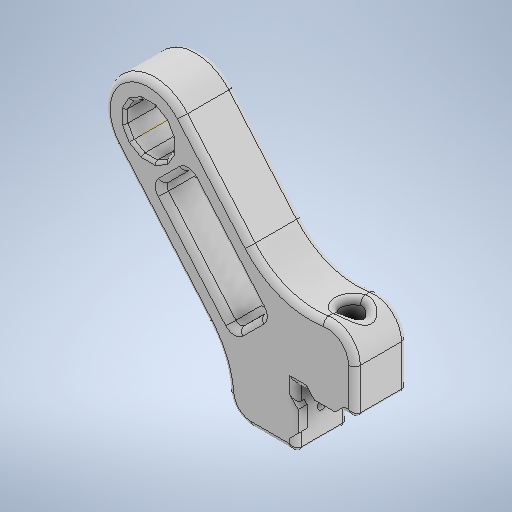
# Autodesk Inventor part: Z-Endstop
Saved by Autodesk Inventor 2025.3 (Build 293356030, 356C)
## iProperties
Created: 2025-10-01
Part Number: Z-Endstop
Material: Generic
Document SubType Name: Modeling
Designer: tvoko
Density: 1 g/cm^3
Appearance: Default
Author: tvoko
Autodesk Inventor part; units mm, degrees
ref_plane "YZ Plane" through (0, 0, 0) normal (1, 0, 0) x (0, 1, 0)
ref_plane "XZ Plane" through (0, 0, 0) normal (0, 1, 0) x (-1, 0, 0)
ref_plane "XY Plane" through (0, 0, 0) normal (0, 0, 1) x (1, 0, 0)
sketch "Sketch1" plane through (0, 0, 0) normal (0, 0, 1) x (1, 0, 0)
  line L0 (-10.05, 10.05) -> (10.05, 10.05)
  line L1 (10.05, 10.05) -> (10.05, -10.05)
  line L2 (10.05, -10.05) -> (-10.05, -10.05)
  line L3 (-10.05, -10.05) -> (-10.05, 10.05)
  line L4 (0, 10.05) -> (0, -10.05) construction
  line L5 (-10.05, 0) -> (10.05, 0) construction
  line L6 (-10.05, 4.5) -> (-9.05, 3.5)
  line L7 (-9.05, 3.5) -> (-9.05, -3.5)
  line L8 (-9.05, -3.5) -> (-10.05, -4.5)
  line L9 (-4.5, 10.05) -> (-3.5, 9.05)
  line L10 (-3.5, 9.05) -> (3.5, 9.05)
  line L11 (3.5, 9.05) -> (4.5, 10.05)
  line L12 (10.05, 10.05) -> (10.05, 25.05)
  line L13 (-10.05, -10.05) -> (-25.05, -10.05)
  line L14 (-25.05, -10.05) -> (-25.05, 10.05)
  line L15 (-9.95, 25.05) -> (-25.05, 10.05)
  line L16 (10.05, 25.05) -> (-9.95, 25.05)
  line L17 (-9.95, 25.05) -> (-9.95, 10.05)
  line L18 (-10.05, 9.95) -> (-25.05, 9.95)
  circle A0 centre (-60, 60) radius 7.95 construction
  arc A1 (-48.653453, 69.811007) -> (-71.346547, 50.188993) centre (-60, 60) ccw
  line L19 (-48.653453, 69.811007) -> (-25.647611, 43.204476)
  line L20 (-71.346547, 50.188993) -> (-39.889181, 13.808171)
  line L21 (-31.969587, 6.010347) -> (-25.05, -10.05) construction
  line L22 (-9.95, 25.05) -> (-31.969587, 6.010347) construction
  line L23 (-9.95, 25.05) -> (-0.739164, 34.199837) construction
  arc A2 (10.05, 25.05) -> (-0.739164, 34.199837) centre (0.775622, 25.05) ccw
  arc A3 (-25.647611, 43.204476) -> (-0.739164, 34.199837) centre (-5.162352, 60.917444) ccw
  line L24 (-25.647611, 43.204476) -> (-9.95, 25.05) construction
  line L25 (-55.410065, 67.95) -> (-50.820131, 60)
  line L26 (-50.820131, 60) -> (-55.410065, 52.05)
  line L27 (-55.410065, 52.05) -> (-64.589935, 52.05)
  line L28 (-64.589935, 52.05) -> (-69.179869, 60)
  line L29 (-69.179869, 60) -> (-64.589935, 67.95)
  line L30 (-64.589935, 67.95) -> (-55.410065, 67.95)
  line L31 (-60, 69.179869) -> (-52.05, 64.589935)
  line L32 (-52.05, 64.589935) -> (-52.05, 55.410065)
  line L33 (-52.05, 55.410065) -> (-60, 50.820131)
  line L34 (-60, 50.820131) -> (-67.95, 55.410065)
  line L35 (-67.95, 55.410065) -> (-67.95, 64.589935)
  line L36 (-67.95, 64.589935) -> (-60, 69.179869)
  line L37 (-47.974498, 53.52563) -> (-55.086003, 46.461221)
  line L38 (-55.189369, 43.734182) -> (-32.242214, 17.195522)
  line L39 (-29.319833, 17.084752) -> (-22.208328, 24.149161)
  line L40 (-22.104962, 26.8762) -> (-45.052118, 53.41486)
  arc A4 (-45.052118, 53.41486) -> (-47.974498, 53.52563) centre (-46.564991, 52.106726) ccw
  arc A5 (-22.208328, 24.149161) -> (-22.104962, 26.8762) centre (-23.617835, 25.568065) ccw
  arc A6 (-32.242214, 17.195522) -> (-29.319833, 17.084752) centre (-30.729341, 18.503656) ccw
  arc A7 (-55.086003, 46.461221) -> (-55.189369, 43.734182) centre (-53.676496, 45.042317) ccw
  arc A8 (-32.932093, -2.78299) -> (-39.889181, 13.808171) centre (-61.791846, -5.130384) ccw
  arc A9 (-32.932093, -2.78299) -> (-25.05, -10.05) centre (-25.05, -2.141876) ccw
  point P0 (0, 0)
  point P1 (0, 0)
  point P2 (0, 9.05)
  point P3 (-9.05, 0)
  point P4 (-60, 67.95)
  point P5 (-63.975, 66.884902)
  point P6 (-52.05, 62.130196)
  point P7 (-52.05, 57.869804)
  point P8 (-54.180196, 54.180196)
  point P9 (-57.869804, 52.05)
  point P10 (-62.130196, 52.05)
  point P11 (-65.819804, 54.180196)
  point P12 (-67.95, 57.869804)
  point P13 (-67.95, 62.130196)
  point P14 (-57.869804, 67.95)
  point P15 (-54.180196, 65.819804)
  point P16 (-65.819804, 65.819804)
  point P17 (-62.130196, 67.95)
  dimension "d0" = 20.1
  dimension "d1" = 7
  dimension "d2" = 1
  dimension "d3" = 135
  dimension "d4" = 1
  dimension "d5" = 7
  dimension "d6" = 135
  dimension "d8" = 15
  dimension "d9" = 15
  dimension "d18" = 20
  dimension "d19" = 20
  dimension "d62" = 60
  dimension "d63" = 15.9
  dimension "d64" = 30
  dimension "d65" = 24
  dimension "d72" = 2
  dimension "d73" = 8
  dimension "d75" = 8
  dimension "d76" = 8
  dimension "d77" = 39
  dimension "d80" = 60
  constraints: 83 end point, 20 point on circle, 16 tangent, 10 centre point, 9 midpoint, 9 point on line, 7 parallel, 7 perpendicular, 5 horizontal, 4 coincident, 4 equal length, 3 equal radius, 2 vertical, 1 collinear, 26 other
  measures "d0" distance of L0.start L0.end
  measures "d1" distance of L9.end L10.end
  measures "d2" distance between parallel lines of L0 L10
  measures "d3" angle of L10 L11
  measures "d4" distance between parallel lines of L3 L7
  measures "d5" distance of L6.end L7.end
  measures "d6" angle of L7 L6
  measures "d8" distance of L2.end L13.end
  measures "d9" distance of L0.end L12.end
  measures "d18" distance of L12.end L15.start
  measures "d19" distance between parallel lines of L13 L18
  measures "d62" distance from line of A0.centre L5
  measures "d63" diameter of A0
  measures "d64" diameter of A1
  measures "d65" distance of L19.end L15.start
  measures "d72" radius of A4
  measures "d73" distance between parallel lines of L19 L40
  measures "d75" distance between parallel lines of L20 L38
  measures "d76" distance between parallel lines of L15 L39
  measures "d77" distance between parallel lines of L39 L37
  measures "d80" distance from line of L4 A0.centre
extrude "Extrusion1" add sketch "Sketch1" along normal mid plane 18 contours L3 L18 L14 L15 L17 L0 | L17 L16 L12 L0 | L3 L13 L14 L18 | L0 L11 L10 L9 | L15 L14 A9 A8 L20 A1 L19 A3 A2 L16 | L6 L7 L8 L3 | L25 L31 L30 | L31 L32 L25 | L30 L36 L31 | L25 L26 L32 | L36 L29 L30 | L32 L33 L26 | L29 L35 L36 | L26 L27 L33 | L35 L28 L29 | L33 L34 L27 | L28 L34 L35 | L27 L28 L34
fillet "Fillet1" radius 1 2 edges at (10.05, 10.05, 0) (-10.05, -10.05, 0)
sketch "Sketch2" plane through (-4.5, 9.05, -9) normal (0, -1, 0) x (-1, 0, 0)
  line L0 (-9, -18) -> (-13.55, -18) projected
  line L1 (-9, 0) -> (-9, -18) projected
  line L2 (0, 0) -> (0, -18) projected
  circle A0 centre (-4.5, -9) radius 1.55
  circle A1 centre (-4.5, -9) radius 3.5
  line L3 (5.55, 0) -> (5.55, -18) projected
  line L4 (0, 0) -> (5.55, 0) projected
  line L5 (-8, 0) -> (-1, 0) projected
  line L6 (-13.55, 0) -> (-9, 0) projected
  line L7 (-13.55, -18) -> (-13.55, 0) projected
  line L8 (5.55, -18) -> (0, -18) projected
  line L9 (-9, -9) -> (0, -9) construction
  line L10 (-9, -15) -> (0, -15)
  line L11 (0, -15) -> (0, -3)
  line L12 (0, -3) -> (-9, -3)
  line L13 (-9, -3) -> (-9, -15)
  point P0 (-4.5, -9)
  point P1 (-1, 0)
  point P2 (0, -15)
  dimension "d26" = 3.1
  dimension "d27" = 7
  dimension "d66" = 12
  constraints: 10 end point, 4 midpoint, 2 centre point, 2 coincident, 2 parallel, 2 point on line, 1 horizontal, 1 perpendicular, 1 other
  measures "d26" diameter of A0
  measures "d27" diameter of A1
  measures "d66" distance between parallel lines of L12 L10
extrude "Extrusion3" cut sketch "Sketch2" against normal through all contours A0 | A1
sketch "Sketch3" plane through (-9.05, -4.5, -9) normal (1, 0, 0) x (0, 0, 1)
  line L0 (0, -14.55) -> (0, -9) projected
  line L1 (18, -9) -> (18, -14.55) projected
  line L2 (0, -9) -> (18, -9) projected
  line L3 (0, 0) -> (18, 0) projected
  circle A0 centre (9, -4.5) radius 3.5
  circle A1 centre (9, -4.5) radius 1.55
  line L4 (0, -14.55) -> (18, -14.55) projected
  line L5 (18, 4.55) -> (18, 0) projected
  line L6 (0, -8) -> (0, -1) projected
  line L7 (9, -9) -> (9, 0) construction
  line L8 (0, 4.55) -> (18, 4.55) projected
  line L9 (0, 0) -> (0, 4.55) projected
  line L10 (0, -9) -> (18, -9) projected
  line L11 (0, 0) -> (18, 0) projected
  line L12 (15, -9) -> (3, -9)
  line L13 (3, -9) -> (3, 0)
  line L14 (3, 0) -> (15, 0)
  line L15 (15, 0) -> (15, -9)
  point P0 (9, -4.5)
  point P1 (0, -1)
  point P2 (15, 0)
  point P3 (3, 0)
  point P4 (3, -9)
  dimension "d30" = 7
  dimension "d31" = 3.1
  dimension "d69" = 12
  constraints: 10 end point, 5 midpoint, 2 centre point, 2 coincident, 2 parallel, 2 point on line, 1 horizontal, 1 perpendicular, 1 other
  measures "d30" diameter of A0
  measures "d31" diameter of A1
  measures "d69" distance between parallel lines of L13 L15
extrude "Extrusion4" cut sketch "Sketch3" against normal through all contours A0 | A1
extrude "Extrusion5" add sketch "Sketch2" against normal blind 4 contours A1
extrude "Extrusion6" add sketch "Sketch3" against normal blind 4 contours A0
extrude "Extrusion9" cut sketch "Sketch2" against normal up to surface (1 mm away) contours L1 L12 L2 L10 | A1
extrude "Extrusion10" cut sketch "Sketch3" against normal up to surface (1 mm away) contours L13 L3 L15 L2 | A0
fillet "Fillet5" radius 2 47 edges at (-25.05, -10.05, 0) (-21.6193, 25.4923, -9) (-33.5785, 40.1455, -9) (-46.4892, 54.1053, -9) (-51.5303, 49.9934, -9) (-55.6751, 45.1181, -9) (-43.7158, 30.4649, -9) (-30.8051, 16.5051, -9) (-25.7641, 20.617, -9) (-55.6751, 45.1181, 9) (-51.5303, 49.9934, 9) (-46.4892, 54.1053, 9) (-33.5785, 40.1455, 9) (-21.6193, 25.4923, 9) (-25.7641, 20.617, 9) (-30.8051, 16.5051, 9) (-43.7158, 30.4649, 9) (-14.3693, 35.4493, -9) (6.7742, 32.1233, -9) (10.05, 18.05, -9) (9.7571, 10.3429, -9) (6.775, 10.05, -9) (-69.811, 71.3465, -9) (-55.6179, 31.9986, -9) (-37.1505, 56.5077, -9) (-69.811, 71.3465, 9) (-55.6179, 31.9986, 9) (-14.3693, 35.4493, 9) (6.7742, 32.1233, 9) (10.05, 18.05, 9) (9.7571, 10.3429, 9) (6.775, 10.05, 9) (-37.1505, 56.5077, 9) (-7.275, 10.05, -9) (-10.05, 7.275, -9) (-10.3429, -9.7571, -9) (-18.05, -10.05, -9) (-10.05, -6.775, -9) (-10.3429, -9.7571, 9) (-10.05, -6.775, 9) (-18.05, -10.05, 9) (-10.05, 7.275, 9) (-7.275, 10.05, 9) (-2.8414, 33.9358, 2.0436) (-2.8414, 33.9358, -2.0436) (3.5, 33.9152, 0.002) (-32.8406, -3.5, -0.0002)
fillet "Fillet6" radius 1 24 edges at (-66.8849, 63.975, -9) (-63.975, 66.8849, -9) (-60, 67.95, -9) (-56.025, 66.8849, -9) (-53.1151, 63.975, -9) (-52.05, 60, -9) (-53.1151, 56.025, -9) (-56.025, 53.1151, -9) (-60, 52.05, -9) (-63.975, 53.1151, -9) (-66.8849, 56.025, -9) (-67.95, 60, -9) (-60, 67.95, 9) (-63.975, 66.8849, 9) (-66.8849, 63.975, 9) (-67.95, 60, 9) (-66.8849, 56.025, 9) (-63.975, 53.1151, 9) (-60, 52.05, 9) (-56.025, 53.1151, 9) (-53.1151, 56.025, 9) (-52.05, 60, 9) (-53.1151, 63.975, 9) (-56.025, 66.8849, 9)
body "Solid1"
